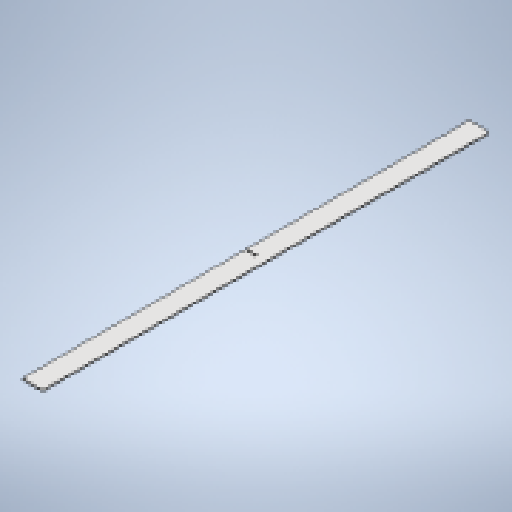
# Autodesk Inventor part: BSH 506 amplifier
Saved by Autodesk Inventor 2025 (Build 290162010, 162A)
## iProperties
Created: 2024-09-03
Part Number: BSH 506 amplifier
Material: Stainless Steel
Document SubType Name: Sheet Metal
Designer: pokla
Density: 8 g/cm^3
Sheet Metal Rule: AISI304 3mm Die 32
Sheet Metal Width: 0,000 mm
Sheet Metal Length: 0,000 mm
Sheet Metal Area: 0,000 mm^2
Appearance: Default
Author: pokla
Autodesk Inventor part; units mm, degrees
ref_plane "YZ Plane" through (0, 0, 0) normal (1, 0, 0) x (0, 1, 0)
ref_plane "XZ Plane" through (0, 0, 0) normal (0, 1, 0) x (-1, 0, 0)
ref_plane "XY Plane" through (0, 0, 0) normal (0, 0, 1) x (1, 0, 0)
sketch "Sketch1" plane through (0, 0, 0) normal (0, 0, 1) x (1, 0, 0)
  line L0 (-25, -549) -> (25, -549)
  line L1 (25, -549) -> (25, 549)
  line L2 (25, 549) -> (-25, 549)
  line L3 (-25, 549) -> (-25, -549)
  line L4 (-25, -549) -> (-25, -511.3932)
  line L5 (-25, -549) -> (25, 549) construction
  line L6 (-25, -1.5) -> (1, -1.5)
  line L7 (1, -1.5) -> (1, 1.5)
  line L8 (1, 1.5) -> (-25, 1.5)
  line L9 (-25, 1.5) -> (-25, -1.5)
  point P0 (0, 0)
  point P1 (0, 0)
  point P2 (-25, 0)
  dimension "d17" = 1098
  dimension "d18" = 50
  dimension "d19" = 3
  dimension "d20" = 26
  measures "d17" distance of L2.end L0.start
  measures "d18" distance of L1.end L2.end
  measures "d19" distance between parallel lines of L6 L8
  measures "d20" distance of L7.end L8.end
extrude "Plate2" add sketch "Sketch1" against normal blind 3 contours L3 L6 L7 L8 L2 L1 L0
fillet "Corner Round2" radius 6 2 edges at (25, -549, -1.5) (25, 549, -1.5)
equation "\"d18\" = Ширина_креста"
equation "\"d19\" = Thickness"
equation "\"d15\" = Thickness"
equation "\"BendReliefWidth\" = Thickness"
equation "\"BendReliefDepth\" = 0.5 * Thickness"
equation "\"CornerReliefSize\" = 4 * Thickness"
equation "\"MinimumRemnant\" = 2 * Thickness"
equation "\"TransitionRadius\" = BendRadius"
equation "\"JacobiRadiusSize\" = BendRadius"
equation "\"GapSize\" = Thickness"
equation "\"Ширина_креста\" = 50"
equation "\"Thickness\" = 3"
equation "\"BendRadius\" = 5"
body "Solid2"
